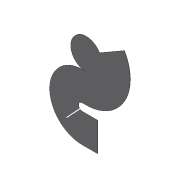
# Autodesk Inventor part: ShooterSketch
Saved by Autodesk Inventor 2012 (Build 160160000, 160)
## iProperties
Created: 2012-01-17
Part Number: ShooterSketch
Material: Default
Document SubType Name: Modeling
Designer: JesseK
Density: 8.64685e-05 g/cm^3
Mass: 0.0453592 g
Surface Area: 4198.99 cm^2
Volume: 524.575 cm^3
Author: JesseK
Autodesk Inventor part; units mm, degrees
ref_plane "YZ Plane" through (0, 0, 0) normal (1, 0, 0) x (0, 1, 0)
ref_plane "XZ Plane" through (0, 0, 0) normal (0, 1, 0) x (-1, 0, 0)
ref_plane "XY Plane" through (0, 0, 0) normal (0, 0, 1) x (1, 0, 0)
sketch "Sketch1" plane through (0, 0, 0) normal (0, 0, 1) x (1, 0, 0)
  arc A0 (368.3, 596.9) -> (621.266, 1035.05) centre (368.3, 889) ccw
  circle A1 centre (368.3, 889) radius 101.6
  line L0 (621.266, 1035.05) -> (368.3, 889) construction
  line L1 (456.2882, 939.8) -> (14.5272, 1704.9525) construction
  line L2 (456.2882, 939.8) -> (-427.2338, 939.8) construction
  line L3 (368.3, 889) -> (368.3, 596.9) construction
  line L4 (368.3, 596.9) -> (342.9, 596.9)
  line L5 (342.9, 596.9) -> (342.9, 787.4) construction
  line L6 (342.9, 787.4) -> (368.3, 787.4)
  line L7 (0, 0) -> (685.8, 0) construction
  line L8 (685.8, 0) -> (685.8, 1498.6) construction
  line L9 (685.8, 1498.6) -> (0, 1498.6) construction
  line L10 (0, 1498.6) -> (0, 0) construction
  line L11 (241.3, 0) -> (444.5, 0) construction
  line L12 (444.5, 0) -> (444.5, 558.8) construction
  line L13 (444.5, 558.8) -> (241.3, 558.8) construction
  line L14 (241.3, 558.8) -> (241.3, 0) construction
  line L15 (241.3, 135.2277) -> (0, 135.2277) construction
  line L16 (444.5, 135.2277) -> (685.8, 135.2277) construction
  line L17 (456.2882, 939.8) -> (621.266, 1035.05)
  arc A2 (342.9, 596.9) -> (342.9, 546.1) centre (342.9, 571.5) ccw
  arc A3 (342.9, 787.4) -> (342.9, 355.6) centre (342.9, 571.5) ccw
  line L18 (342.9, 546.1) -> (444.5, 546.1)
  line L19 (342.9, 355.6) -> (444.5, 355.6)
  line L20 (444.5, 355.6) -> (444.5, 546.1)
  arc A4 (342.9, 787.4) -> (343.2908, 790.5262) centre (342.9, 788.9875) ccw
  circle A5 centre (342.9, 571.5) radius 25.4
  line L21 (323.3933, 555.232) -> (232.8369, 458.0957)
  line L22 (237.4816, 453.7656) -> (232.8369, 458.0957)
  line L23 (237.4816, 453.7656) -> (328.038, 550.9019)
  line L24 (328.038, 550.9019) -> (323.3933, 555.232)
  line L25 (357.762, 592.0981) -> (448.3184, 689.2344)
  line L26 (448.3184, 689.2344) -> (452.9631, 684.9043)
  line L27 (452.9631, 684.9043) -> (362.4067, 587.768)
  line L28 (362.4067, 587.768) -> (357.762, 592.0981)
  dimension "d0" = 203.2
  dimension "d2" = 60
  dimension "d3" = 120
  dimension "d5" = 685.8
  dimension "d6" = 1498.6
  dimension "d7" = 203.2
  dimension "d8" = 558.8
  dimension "d9" = 190.5
  dimension "d14" = 25.4
  dimension "d15" = 939.8
  dimension "d21" = 25.4
  dimension "d22" = 101.6
  dimension "d25" = 6.35
  constraints: 58 end point, 18 point on circle, 7 horizontal, 7 parallel, 6 centre point, 6 perpendicular, 6 point on line, 6 tangent, 5 equal length, 4 collinear, 3 coincident, 1 vertical
  measures "d0" diameter of A1
  measures "d2" angle of L2 L1
  measures "d3" angle of L3 L0
  measures "d5" distance between parallel lines of L10 L8
  measures "d6" distance of L9.end L7.start
  measures "d7" distance of L12.end L13.end
  measures "d8" distance between parallel lines of L11 L13
  measures "d9" radial gap between concentric circles of A0 A1
  measures "d14" radius of A2
  measures "d15" distance between parallel lines of L7 L2
  measures "d21" distance of L3.end L4.end
  measures "d22" distance from line of L20 A2.centre
  measures "d25" distance of L27.end L25.start
extrude "Extrusion2" add sketch "Sketch1" along normal blind 2.54 contours L4 L25 L26 L27 A0 | L27 L26 L25 L4 A2 L21 L22 L23 L18 L20 L19 A3 L6 A1 L17 A0 | A1
body "Solid2"
